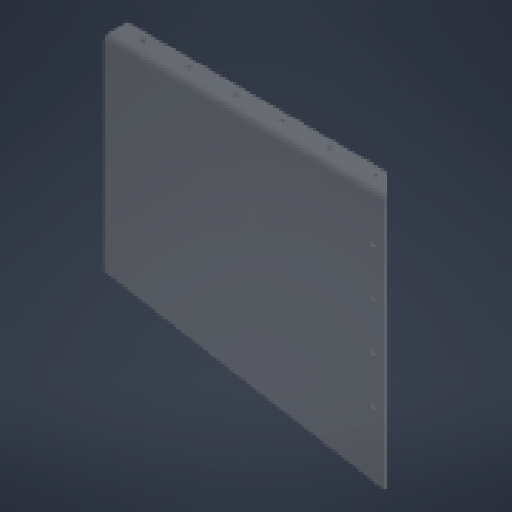
# Autodesk Inventor part: SIDE_INTAKE_LEXAN
Saved by Autodesk Inventor 2026.2 (Build 302298010, 298A)
## iProperties
Created: 2026-04-02
Part Number: SIDE_INTAKE_LEXAN
Material: Polycarbonate, PC 1000, Clear
Document SubType Name: Sheet Metal
Designer: 4aida
Density: 1.20131 g/cm^3
Sheet Metal Rule: Default_mm
Appearance: Lexan (Clear)
Author: 4aida
Autodesk Inventor part; units mm, degrees
ref_plane "YZ Plane" through (0, 0, 0) normal (1, 0, 0) x (0, 1, 0)
ref_plane "XZ Plane" through (0, 0, 0) normal (0, 1, 0) x (-1, 0, 0)
ref_plane "XY Plane" through (0, 0, 0) normal (0, 0, 1) x (1, 0, 0)
sketch "Sketch1" plane through (0, 0, 0) normal (1, 0, 0) x (0, 1, 0)
  line L0 (0, 0) -> (276.225, 0)
  line L1 (276.225, 0) -> (276.225, -25.4)
  dimension "d0" = 25.4
  dimension "d1" = 276.225
  measures "d0" distance of L0.end L1.end
  measures "d1" distance of L0.start L0.end
contour flange "Contour Flange1" sketch "Sketch1" thickness 3.175 bend radius 3.175 width 304.8 along (1, 0, 0) mid plane no both sides no wall seen from (0, 138.1125, 0) lies toward (0, 0, -1) curves L0 L1
bend "Bend1"
corner "Corner1"
sketch "Sketch2" plane through (0, 0, 0) normal (0, 0, 1) x (1, 0, 0)
  line L0 (304.8, 0) -> (304.8, 269.875) projected
  line L1 (304.8, 0) -> (0, 53.7445)
  line L2 (0, 0) -> (0, 269.875) projected
  line L3 (0, 269.875) -> (304.8, 269.875) projected
  line L4 (0, 0) -> (0, 269.875) projected
  line L5 (304.8, 0) -> (0, 0) projected
  line L6 (304.8, 269.875) -> (304.8, 0) projected
  dimension "d13" = 10
  constraints: 2 end point, 1 point on line
  measures "d13" angle of L1 L5
extrude "Cut1" cut sketch "Sketch2" against normal blind 3.175 contours L5 L2 L1
sketch "Sketch3" plane through (0, 276.225, -25.4) normal (0, 1, 0) x (1, 0, 0)
  line L0 (304.8, -22.225) -> (282.575, 0)
  line L1 (0, 0) -> (304.8, 0) projected
  line L2 (304.8, 0) -> (304.8, -19.05) projected
  line L3 (304.8, 0) -> (304.8, -22.225)
  point P0 (0, -25.4)
  dimension "d16" = 45
  constraints: 4 end point, 1 collinear, 1 point on line
  measures "d16" angle of L2 L0
extrude "Cut2" cut sketch "Sketch3" against normal through all
sketch "Sketch4" plane through (0, 269.875, 0) normal (0, 0, 1) x (1, 0, 0)
  line L0 (304.8, 0) -> (304.8, -269.875) projected
  point P0 (0, -269.875)
  point P1 (292.1, -196.85)
  point P2 (292.1, -146.05)
  point P3 (292.1, -95.25)
  point P4 (292.1, -44.45)
  dimension "d19" = 73.025
  dimension "d20" = 12.7
  dimension "d23" = 50.8
  constraints: 1 vertical, 3 other
  measures "d19" vertical distance of L0.end point (292.1, -196.85)
  measures "d20" distance from line of L0 point (292.1, -196.85)
  measures "d23" distance of point (292.1, -196.85) point (292.1, -146.05)
hole "Hole1" at (292.1, 73.025, 0) at (292.1, 123.825, 0) at (292.1, 174.625, 0) at (292.1, 225.425, 0) direction (0, 0, -1) diameter 5.105 end through all clearance for "Flat Head Machine Screw (82)" size "#10" standard "Ansi Unified Screw Threads"
sketch "Sketch5" plane through (0, 276.225, -6.35) normal (0, 1, 0) x (1, 0, 0)
  line L0 (0, 19.05) -> (282.575, 19.05) projected
  line L1 (0, 0) -> (0, 19.05) projected
  point P0 (0, -6.35)
  point P1 (25.4, 9.525)
  point P2 (76.2, 9.525)
  point P3 (127, 9.525)
  point P4 (177.8, 9.525)
  point P5 (228.6, 9.525)
  point P6 (279.4, 9.525)
  dimension "d35" = 9.525
  dimension "d36" = 25.4
  dimension "d39" = 50.8
  constraints: 1 horizontal, 5 other
  measures "d35" distance from line of L0 point (25.4, 9.525)
  measures "d36" distance from line of L1 point (25.4, 9.525)
  measures "d39" distance of point (25.4, 9.525) point (76.2, 9.525)
hole "Hole2" at (25.4, 276.225, -15.875) at (76.2, 276.225, -15.875) at (127, 276.225, -15.875) at (177.8, 276.225, -15.875) at (228.6, 276.225, -15.875) at (279.4, 276.225, -15.875) direction (0, -1, 0) diameter 5.105 end through all clearance for "Flat Head Machine Screw (82)" size "#10" standard "Ansi Unified Screw Threads"
equation "\"d14\" = Thickness"
equation "\"d17\" = Thickness"
equation "\"d33\" = Thickness"
equation "\"d2\" = Thickness"
equation "\"d3\" = BendReliefWidth"
equation "\"d4\" = BendReliefDepth"
equation "\"d5\" = MinimumRemnant"
equation "\"d6\" = TransitionRadius"
equation "\"d8\" = BendRadius"
equation "\"d10\" = CornerReliefSize"
equation "\"d11\" = GapSize"
equation "\"d12\" = JacobiRadiusSize"
equation "\"BendRadius\" = Thickness"
equation "\"BendReliefWidth\" = Thickness"
equation "\"BendReliefDepth\" = 0.5 * Thickness"
equation "\"CornerReliefSize\" = 4 * Thickness"
equation "\"MinimumRemnant\" = 2 * Thickness"
equation "\"TransitionRadius\" = BendRadius"
equation "\"JacobiRadiusSize\" = BendRadius"
equation "\"GapSize\" = Thickness"
equation "\"Thickness\" = 3.175"
body "Solid1"
